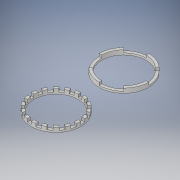
# Autodesk Inventor part: contadores circulares
Saved by Autodesk Inventor 2019.4 (Build 234330000, 330)
## iProperties
Created: 2019-11-21
Part Number: contadores circulares
Material: Genérico
Document SubType Name: Modeling
Designer: natha
Density: 1 g/cm^3
Appearance: Padrão
Author: natha
Autodesk Inventor part; units mm, degrees
ref_plane "YZ Plane" through (0, 0, 0) normal (1, 0, 0) x (0, 1, 0)
ref_plane "XZ Plane" through (0, 0, 0) normal (0, 1, 0) x (-1, 0, 0)
ref_plane "XY Plane" through (0, 0, 0) normal (0, 0, 1) x (1, 0, 0)
sketch "Esboço1" plane through (0, 0, 0) normal (0, 1, 0) x (-1, 0, 0)
  circle A0 centre (0, 0) radius 24.5
  circle A1 centre (0, 0) radius 27.5
  dimension "d0" = 49
  dimension "d1" = 55
  constraints: 2 centre point, 2 coincident
  measures "d0" diameter of A0
  measures "d1" diameter of A1
extrude "Extrusão1" add sketch "Esboço1" along normal blind 2
sketch "Esboço2" plane through (0, 2, 0) normal (0, 1, 0) x (1, 0, 0)
  arc A0 (-19.4454, 19.4454) -> (-27.5, 0) centre (0, 0) ccw
  line L0 (0, 0) -> (-19.4454, 19.4454) construction
  line L1 (0, 0) -> (-27.5, 0) construction
  arc A1 (-17.3241, 17.3241) -> (-24.5, 0) centre (0, 0) ccw
  line L2 (0, 0) -> (-17.3241, 17.3241) construction
  line L3 (0, 0) -> (-24.5, 0) construction
  line L4 (-17.3241, 17.3241) -> (-19.4454, 19.4454)
  line L5 (-27.5, 0) -> (-24.5, 0)
  arc A2 (-17.3241, -17.3241) -> (0, -24.5) centre (0, 0) ccw
  arc A3 (-19.4454, -19.4454) -> (0, -27.5) centre (0, 0) ccw
  line L6 (0, 0) -> (0, -27.5) construction
  line L7 (0, -27.5) -> (0, -24.5)
  line L8 (-17.3241, -17.3241) -> (-19.4454, -19.4454)
  arc A4 (17.3241, -17.3241) -> (24.5, 0) centre (0, 0) ccw
  arc A5 (19.4454, -19.4454) -> (27.5, 0) centre (0, 0) ccw
  line L9 (0, 0) -> (27.5, 0) construction
  line L10 (27.5, 0) -> (24.5, 0)
  line L11 (17.3241, -17.3241) -> (19.4454, -19.4454)
  arc A6 (17.3241, 17.3241) -> (0, 24.5) centre (0, 0) ccw
  arc A7 (19.4454, 19.4454) -> (0, 27.5) centre (0, 0) ccw
  line L12 (0, 0) -> (0, 27.5) construction
  line L13 (0, 27.5) -> (0, 24.5)
  line L14 (17.3241, 17.3241) -> (19.4454, 19.4454)
  dimension "d4" = 45
  dimension "d5" = 45
  dimension "d8" = 360
  constraints: 30 end point, 16 point on circle, 8 centre point, 2 coincident, 1 collinear, 45 other
  measures "d4" angle of L0 L1
  measures "d5" angle of L2 L3
extrude "Extrusão2" add sketch "Esboço2" along normal blind 3
sketch "Esboço4" plane through (0, 0, 0) normal (0, 1, 0) x (-1, 0, 0)
  circle A0 centre (0, 75.0604) radius 24.5
  circle A1 centre (0, 75.0604) radius 27.5
  point P0 (0, 0)
  dimension "d12" = 49
  dimension "d13" = 55
  constraints: 2 centre point, 1 coincident
  measures "d12" diameter of A0
  measures "d13" diameter of A1
extrude "Extrusão3" add sketch "Esboço4" along normal blind 2
sketch "Esboço5" plane through (0, 2, 75.0604) normal (0, 1, 0) x (1, 0, 0)
  arc A0 (-27.0822, 4.7753) -> (-27.5, 0) centre (0, 0) ccw
  line L0 (0, 0) -> (-27.0822, 4.7753) construction
  line L1 (0, 0) -> (-27.5, 0) construction
  arc A1 (-24.1278, 4.2544) -> (-24.5, 0) centre (0, 0) ccw
  line L2 (-27.5, 0) -> (-24.5, 0)
  line L3 (-27.0822, 4.7753) -> (-24.1278, 4.2544)
  line L4 (0, 0) -> (-25.8415, -9.4056) construction
  line L5 (-25.8415, -9.4056) -> (-23.0225, -8.3795)
  line L6 (-27.0822, -4.7753) -> (-24.1278, -4.2544)
  arc A2 (-27.0822, -4.7753) -> (-25.8415, -9.4056) centre (0, 0) ccw
  arc A3 (-24.1278, -4.2544) -> (-23.0225, -8.3795) centre (0, 0) ccw
  line L7 (0, 0) -> (-21.0662, -17.6767) construction
  line L8 (-21.0662, -17.6767) -> (-18.7681, -15.7483)
  line L9 (-23.8157, -13.75) -> (-21.2176, -12.25)
  arc A4 (-23.8157, -13.75) -> (-21.0662, -17.6767) centre (0, 0) ccw
  arc A5 (-21.2176, -12.25) -> (-18.7681, -15.7483) centre (0, 0) ccw
  line L10 (0, 0) -> (-13.75, -23.8157) construction
  line L11 (-13.75, -23.8157) -> (-12.25, -21.2176)
  line L12 (-17.6767, -21.0662) -> (-15.7483, -18.7681)
  arc A6 (-17.6767, -21.0662) -> (-13.75, -23.8157) centre (0, 0) ccw
  arc A7 (-15.7483, -18.7681) -> (-12.25, -21.2176) centre (0, 0) ccw
  line L13 (0, 0) -> (-4.7753, -27.0822) construction
  line L14 (-4.7753, -27.0822) -> (-4.2544, -24.1278)
  line L15 (-9.4056, -25.8415) -> (-8.3795, -23.0225)
  arc A8 (-9.4056, -25.8415) -> (-4.7753, -27.0822) centre (0, 0) ccw
  arc A9 (-8.3795, -23.0225) -> (-4.2544, -24.1278) centre (0, 0) ccw
  line L16 (0, 0) -> (4.7753, -27.0822) construction
  line L17 (4.7753, -27.0822) -> (4.2544, -24.1278)
  line L18 (0, -27.5) -> (0, -24.5)
  arc A10 (0, -27.5) -> (4.7753, -27.0822) centre (0, 0) ccw
  arc A11 (0, -24.5) -> (4.2544, -24.1278) centre (0, 0) ccw
  line L19 (0, 0) -> (13.75, -23.8157) construction
  line L20 (13.75, -23.8157) -> (12.25, -21.2176)
  line L21 (9.4056, -25.8415) -> (8.3795, -23.0225)
  arc A12 (9.4056, -25.8415) -> (13.75, -23.8157) centre (0, 0) ccw
  arc A13 (8.3795, -23.0225) -> (12.25, -21.2176) centre (0, 0) ccw
  line L22 (0, 0) -> (21.0662, -17.6767) construction
  line L23 (21.0662, -17.6767) -> (18.7681, -15.7483)
  line L24 (17.6767, -21.0662) -> (15.7483, -18.7681)
  arc A14 (17.6767, -21.0662) -> (21.0662, -17.6767) centre (0, 0) ccw
  arc A15 (15.7483, -18.7681) -> (18.7681, -15.7483) centre (0, 0) ccw
  line L25 (0, 0) -> (25.8415, -9.4056) construction
  line L26 (25.8415, -9.4056) -> (23.0225, -8.3795)
  line L27 (23.8157, -13.75) -> (21.2176, -12.25)
  arc A16 (23.8157, -13.75) -> (25.8415, -9.4056) centre (0, 0) ccw
  arc A17 (21.2176, -12.25) -> (23.0225, -8.3795) centre (0, 0) ccw
  line L28 (0, 0) -> (27.5, 0) construction
  line L29 (27.5, 0) -> (24.5, 0)
  line L30 (27.0822, -4.7753) -> (24.1278, -4.2544)
  arc A18 (27.0822, -4.7753) -> (27.5, 0) centre (0, 0) ccw
  arc A19 (24.1278, -4.2544) -> (24.5, 0) centre (0, 0) ccw
  line L31 (0, 0) -> (25.8415, 9.4056) construction
  line L32 (25.8415, 9.4056) -> (23.0225, 8.3795)
  line L33 (27.0822, 4.7753) -> (24.1278, 4.2544)
  arc A20 (27.0822, 4.7753) -> (25.8415, 9.4056) centre (0, 0) ccw
  arc A21 (24.1278, 4.2544) -> (23.0225, 8.3795) centre (0, 0) ccw
  line L34 (0, 0) -> (21.0662, 17.6767) construction
  line L35 (21.0662, 17.6767) -> (18.7681, 15.7483)
  line L36 (23.8157, 13.75) -> (21.2176, 12.25)
  arc A22 (23.8157, 13.75) -> (21.0662, 17.6767) centre (0, 0) ccw
  arc A23 (21.2176, 12.25) -> (18.7681, 15.7483) centre (0, 0) ccw
  line L37 (0, 0) -> (13.75, 23.8157) construction
  line L38 (13.75, 23.8157) -> (12.25, 21.2176)
  line L39 (17.6767, 21.0662) -> (15.7483, 18.7681)
  arc A24 (17.6767, 21.0662) -> (13.75, 23.8157) centre (0, 0) ccw
  arc A25 (15.7483, 18.7681) -> (12.25, 21.2176) centre (0, 0) ccw
  line L40 (0, 0) -> (4.7753, 27.0822) construction
  line L41 (4.7753, 27.0822) -> (4.2544, 24.1278)
  line L42 (9.4056, 25.8415) -> (8.3795, 23.0225)
  arc A26 (9.4056, 25.8415) -> (4.7753, 27.0822) centre (0, 0) ccw
  arc A27 (8.3795, 23.0225) -> (4.2544, 24.1278) centre (0, 0) ccw
  line L43 (0, 0) -> (-4.7753, 27.0822) construction
  line L44 (-4.7753, 27.0822) -> (-4.2544, 24.1278)
  line L45 (0, 27.5) -> (0, 24.5)
  arc A28 (0, 27.5) -> (-4.7753, 27.0822) centre (0, 0) ccw
  arc A29 (0, 24.5) -> (-4.2544, 24.1278) centre (0, 0) ccw
  line L46 (0, 0) -> (-13.75, 23.8157) construction
  line L47 (-13.75, 23.8157) -> (-12.25, 21.2176)
  line L48 (-9.4056, 25.8415) -> (-8.3795, 23.0225)
  arc A30 (-9.4056, 25.8415) -> (-13.75, 23.8157) centre (0, 0) ccw
  arc A31 (-8.3795, 23.0225) -> (-12.25, 21.2176) centre (0, 0) ccw
  line L49 (0, 0) -> (-21.0662, 17.6767) construction
  line L50 (-21.0662, 17.6767) -> (-18.7681, 15.7483)
  line L51 (-17.6767, 21.0662) -> (-15.7483, 18.7681)
  arc A32 (-17.6767, 21.0662) -> (-21.0662, 17.6767) centre (0, 0) ccw
  arc A33 (-15.7483, 18.7681) -> (-18.7681, 15.7483) centre (0, 0) ccw
  line L52 (0, 0) -> (-25.8415, 9.4056) construction
  line L53 (-25.8415, 9.4056) -> (-23.0225, 8.3795)
  line L54 (-23.8157, 13.75) -> (-21.2176, 12.25)
  arc A34 (-23.8157, 13.75) -> (-25.8415, 9.4056) centre (0, 0) ccw
  arc A35 (-21.2176, 12.25) -> (-23.0225, 8.3795) centre (0, 0) ccw
  point P0 (0, 75.0604)
  dimension "d16" = 10
  dimension "d19" = 360
  constraints: 110 end point, 72 point on circle, 36 centre point, 19 point on line, 3 coincident, 1 collinear, 1 horizontal, 197 other
  measures "d16" angle of L0 L1
extrude "Extrusão4" add sketch "Esboço5" along normal blind 3
